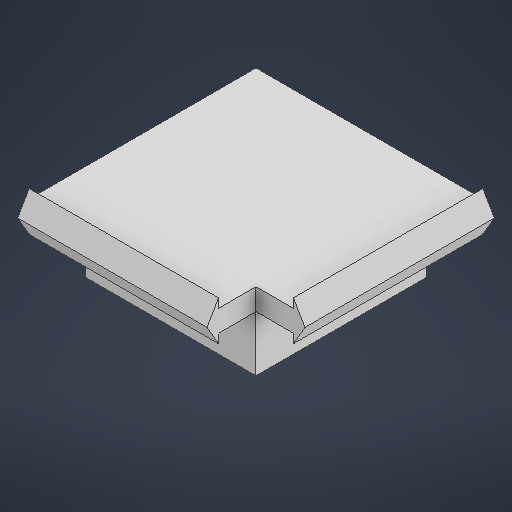
# Autodesk Inventor part: corner support
Saved by Autodesk Inventor 2026.2 (Build 302298000, 298)
## iProperties
Created: 2026-01-08
Part Number: corner support
Material: Generic
Document SubType Name: Modeling
Designer: dongr
Density: 1 g/cm^3
Appearance: Default
Author: dongr
Autodesk Inventor part; units mm, degrees
ref_plane "YZ Plane" through (0, 0, 0) normal (1, 0, 0) x (0, 1, 0)
ref_plane "XZ Plane" through (0, 0, 0) normal (0, 1, 0) x (-1, 0, 0)
ref_plane "XY Plane" through (0, 0, 0) normal (0, 0, 1) x (1, 0, 0)
sketch "Sketch1" plane through (0, 0, 0) normal (0, 1, 0) x (-1, 0, 0)
  line L0 (0, 0) -> (50.8, 0)
  line L1 (50.8, 0) -> (50.8, -50.8)
  line L2 (50.8, -50.8) -> (0, -50.8)
  line L3 (0, -50.8) -> (0, 0)
  dimension "d0" = 50.8
  dimension "d1" = 50.8
  constraints: 8 end point, 2 parallel, 1 horizontal, 1 perpendicular
  measures "d0" distance of L1.end L2.end
  measures "d1" distance of L0.end L1.end
extrude "Extrusion1" add sketch "Sketch1" along normal blind 4.826
sketch "Sketch2" plane through (0, 4.826, 0) normal (0, 1, 0) x (1, 0, 0)
  line L0 (0, 0) -> (-8.382, 0)
  line L1 (-8.382, 0) -> (-8.382, 8.382)
  line L2 (-8.382, 8.382) -> (0, 8.382)
  line L3 (0, 8.382) -> (0, 0)
  line L4 (-8.382, 8.382) -> (-50.8, 8.382)
  line L5 (-50.8, 50.8) -> (-50.8, 0) projected
  line L6 (-8.382, 8.382) -> (-8.382, 50.8)
  dimension "d4" = 8.382
  dimension "d5" = 8.382
  constraints: 12 end point, 2 horizontal, 2 parallel, 1 perpendicular, 1 point on line, 1 vertical
  measures "d4" distance of L1.end L2.end
  measures "d5" distance of L0.end L1.end
extrude "Extrusion2" cut sketch "Sketch2" against normal blind 4.826
sketch "Sketch3" plane through (-8.382, 4.826, 0) normal (1, 0, 0) x (0, 0, -1)
  line L0 (0, -4.826) -> (0, 0) projected
  line L1 (0, 0) -> (0, 2.032)
  line L2 (0, -4.826) -> (0, -6.858)
  line L3 (0, -6.858) -> (-6.204, 3.8876)
  line L4 (0, 2.032) -> (-4.5461, -5.842)
  line L5 (0, 2.032) -> (9.0921, 2.032) construction
  point P0 (-2.5663, -2.413)
  dimension "d8" = 2.032
  dimension "d9" = 2.032
  dimension "d10" = 30
  dimension "d11" = 120
  constraints: 10 end point, 2 vertical, 1 equal length, 1 horizontal
  measures "d8" distance of L0.end L1.end
  measures "d9" distance of L0.start L2.end
  measures "d10" angle of L2 L3
  measures "d11" angle of L4 L5
extrude "Extrusion3" add sketch "Sketch3" against normal blind 42.418
sketch "Sketch4" plane through (-8.382, 4.826, -8.382) normal (0, 0, 1) x (1, 0, 0)
  line L0 (8.382, 0) -> (8.382, 2.032)
  line L1 (8.382, 0) -> (10.414, 0) construction
  line L2 (8.382, -4.826) -> (8.382, -6.858)
  line L3 (8.382, -6.858) -> (14.7819, 4.2269)
  line L4 (8.382, 2.032) -> (14.3676, -8.3353)
  line L5 (8.382, 2.032) -> (20.3531, 2.032) construction
  line L6 (8.382, 0) -> (-42.418, 0) projected
  line L7 (8.382, 0) -> (8.382, -4.826)
  point P0 (10.9483, -2.413)
  dimension "d14" = 2.032
  dimension "d15" = 90
  dimension "d16" = 2.032
  dimension "d17" = 30
  dimension "d18" = 60
  constraints: 14 end point, 2 equal length, 2 horizontal, 2 vertical, 1 perpendicular
  measures "d14" distance of L0.start L0.end
  measures "d15" angle of L1 L0
  measures "d16" distance of L2.start L2.end
  measures "d17" angle of L3 L2
  measures "d18" angle of L4 L5
extrude "Extrusion4" add sketch "Sketch4" against normal blind 42.418
sketch "Sketch6" plane through (0, 0, 0) normal (0, -1, 0) x (1, 0, 0)
  line L0 (-50.8, -50.8) -> (-50.8, 0) projected
  line L1 (-50.8, -50.8) -> (-12.7, -50.8)
  line L2 (-12.7, -50.8) -> (-12.7, -12.7)
  line L3 (-12.7, -12.7) -> (-50.8, -12.7)
  line L4 (-50.8, -12.7) -> (-50.8, -50.8)
  point P0 (0, 0)
  dimension "d21" = 38.1
  dimension "d22" = 38.1
  constraints: 8 end point, 2 parallel, 1 horizontal, 1 perpendicular
  measures "d21" distance of L3.end L2.end
  measures "d22" distance of L2.end L1.end
extrude "Extrusion5" add sketch "Sketch6" along normal blind 16.764
body "Solid1"
